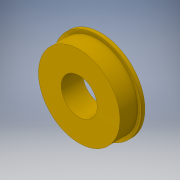
# Autodesk Inventor part: Bearing
Saved by Autodesk Inventor 2016 SP2 (Build 200236200, 236)
## iProperties
Created: 2017-01-16
Part Number: Bearing
Material: Generic
Document SubType Name: Modeling
Designer: CAD
Density: 1 g/cm^3
Appearance: Gold
Author: CAD
Autodesk Inventor part; units mm, degrees
ref_plane "YZ Plane" through (0, 0, 0) normal (1, 0, 0) x (0, 1, 0)
ref_plane "XZ Plane" through (0, 0, 0) normal (0, 1, 0) x (-1, 0, 0)
ref_plane "XY Plane" through (0, 0, 0) normal (0, 0, 1) x (1, 0, 0)
sketch "Sketch1" plane through (0, 0, 0) normal (0, 0, 1) x (1, 0, 0)
  circle A0 centre (0, 0) radius 15.494
  dimension "d0" = 30.988
  constraints: 1 centre point, 1 coincident
  measures "d0" diameter of A0
extrude "Extrusion1" add sketch "Sketch1" along normal blind 1.27
sketch "Sketch2" plane through (0, 0, 1.27) normal (0, 0, 1) x (1, 0, 0)
  circle A0 centre (0, 0) radius 14.2875
  dimension "d3" = 28.575
  constraints: 1 centre point, 1 coincident
  measures "d3" diameter of A0
extrude "Extrusion2" add sketch "Sketch2" along normal blind 6.35
sketch "Sketch3" plane through (0, 0, 7.62) normal (0, 0, 1) x (1, 0, 0)
  point P0 (0, 0)
  point P1 (0, 0)
  constraints: 1 coincident
hole "Hole1" at (0, 0, 7.62) direction (0, 0, -1) diameter 12.7 end through all
body "Solid1"
